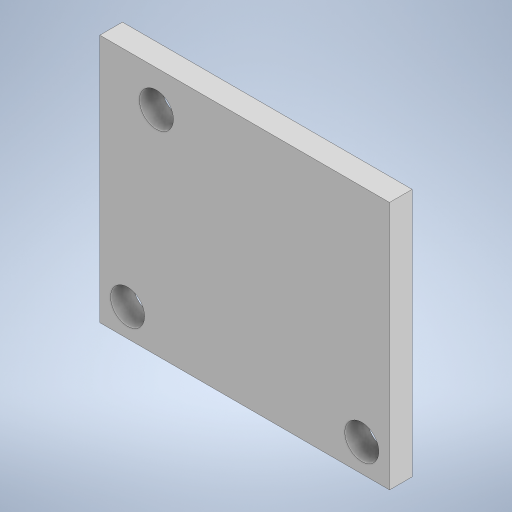
# Autodesk Inventor part: Plate_SEN_Current_sensor
Saved by Autodesk Inventor 2023.1 (Build 271208000, 208)
## iProperties
Created: 2023-01-27
Part Number: Plate_SEN_Current_sensor
Material: Generic
Document SubType Name: Modeling
Designer: Windows10
Density: 1 g/cm^3
Appearance: Default
Author: Windows10
Autodesk Inventor part; units mm, degrees
ref_plane "YZ Plane" through (0, 0, 0) normal (1, 0, 0) x (0, 1, 0)
ref_plane "XZ Plane" through (0, 0, 0) normal (0, 1, 0) x (-1, 0, 0)
ref_plane "XY Plane" through (0, 0, 0) normal (0, 0, 1) x (1, 0, 0)
sketch "Sketch1" plane through (0, 0, 0) normal (0, 0, 1) x (1, 0, 0)
  line L0 (0, 0) -> (25.6, 0)
  line L1 (25.6, 0) -> (25.6, -22)
  line L2 (25.6, -22) -> (0, -22)
  line L3 (0, -22) -> (0, 0)
  circle A0 centre (2.45, -19.55) radius 1.5
  line L4 (12.8, -22) -> (12.8, -20.4874)
  circle A1 centre (23.15, -19.55) radius 1.5
  circle A2 centre (5, -3.2) radius 1.5
  dimension "d0" = 25.6
  dimension "d1" = 22
  dimension "d2" = 3
  dimension "d3" = 2.45
  dimension "d4" = 2.45
  dimension "d5" = 3.2
  dimension "d6" = 3
  constraints: 10 end point, 3 centre point, 2 parallel, 1 horizontal, 1 midpoint, 1 perpendicular, 1 symmetric about line, 1 vertical, 1 other
  measures "d0" distance of L1.end L2.end
  measures "d1" distance of L0.end L1.end
  measures "d2" diameter of A0
  measures "d3" distance from line of L2 A0.centre
  measures "d4" distance from line of L3 A0.centre
  measures "d5" distance from line of L0 A2.centre
  measures "d6" diameter of A2
extrude "Extrusion1" add sketch "Sketch1" along normal blind 2
body "Solid1"
